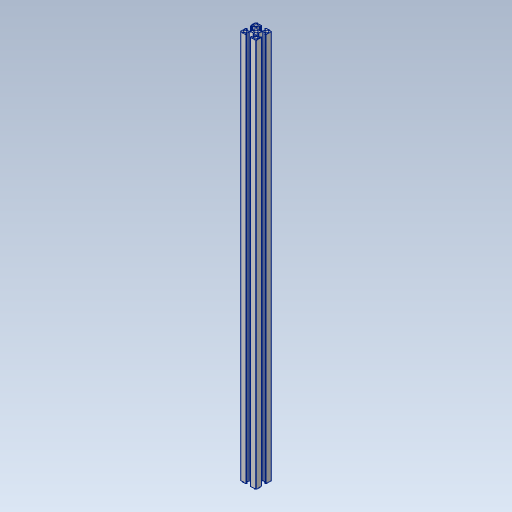
# Autodesk Inventor part: 100mm 2020
Saved by Autodesk Inventor 2021 (Build 250183000, 183)
## iProperties
Created: 2019-12-30
Part Number: 100mm 2020
Material: 알루미늄 6061
Document SubType Name: Modeling
Designer: leejun
Density: 2.7 g/cm^3
Appearance: 알루미늄 - 평지
Author: leejun
Autodesk Inventor part; units mm, degrees
ref_plane "YZ Plane" through (0, 0, 0) normal (1, 0, 0) x (0, 1, 0)
ref_plane "XZ Plane" through (0, 0, 0) normal (0, 1, 0) x (-1, 0, 0)
ref_plane "XY Plane" through (0, 0, 0) normal (0, 0, 1) x (1, 0, 0)
sketch "2020_Base" plane through (0, 0, 0) normal (0, 1, 0) x (-1, 0, 0)
  line L0 (2307.7639, 1192.1343) -> (2307.7639, 1195.3915) projected
  arc A0 (2307.7639, 1195.3915) -> (2307.4639, 1195.6915) centre (2307.4639, 1195.3915) ccw projected
  line L1 (2307.4639, 1195.6915) -> (2306.5639, 1195.6915) projected
  arc A1 (2306.2639, 1195.9915) -> (2306.5639, 1195.6915) centre (2306.5639, 1195.9915) ccw projected
  line L2 (2306.2639, 1195.9915) -> (2306.2639, 1196.8915) projected
  arc A2 (2306.5639, 1197.1915) -> (2306.2639, 1196.8915) centre (2306.5639, 1196.8915) ccw projected
  line L3 (2306.5639, 1197.1915) -> (2313.3139, 1197.1915) projected
  arc A3 (2313.6139, 1196.8915) -> (2313.3139, 1197.1915) centre (2313.3139, 1196.8915) ccw projected
  line L4 (2313.6139, 1196.8915) -> (2313.6139, 1190.1415) projected
  arc A4 (2313.3139, 1189.8415) -> (2313.6139, 1190.1415) centre (2313.3139, 1190.1415) ccw projected
  line L5 (2313.3139, 1189.8415) -> (2312.4139, 1189.8415) projected
  arc A5 (2312.1139, 1190.1415) -> (2312.4139, 1189.8415) centre (2312.4139, 1190.1415) ccw projected
  line L6 (2312.1139, 1190.1415) -> (2312.1139, 1191.0415) projected
  arc A6 (2312.1139, 1191.0415) -> (2311.8139, 1191.3415) centre (2311.8139, 1191.0415) ccw projected
  line L7 (2311.8139, 1191.3415) -> (2308.5567, 1191.3415) projected
  arc A7 (2308.5567, 1191.3415) -> (2308.3217, 1191.2281) centre (2308.5567, 1191.0415) ccw projected
  arc A8 (2308.3217, 1191.2281) -> (2306.9212, 1187.4988) centre (2313.4048, 1187.1915) ccw projected
  line L8 (2306.9212, 1187.4988) -> (2306.6139, 1187.1915) projected
  line L9 (2306.6139, 1187.1915) -> (2306.9212, 1186.8843) projected
  arc A9 (2306.9212, 1186.8843) -> (2308.3217, 1183.155) centre (2313.4048, 1187.1915) ccw projected
  arc A10 (2308.3217, 1183.155) -> (2308.5567, 1183.0415) centre (2308.5567, 1183.3415) ccw projected
  line L10 (2308.5567, 1183.0415) -> (2311.8139, 1183.0415) projected
  arc A11 (2311.8139, 1183.0415) -> (2312.1139, 1183.3415) centre (2311.8139, 1183.3415) ccw projected
  line L11 (2312.1139, 1183.3415) -> (2312.1139, 1184.2415) projected
  arc A12 (2312.4139, 1184.5415) -> (2312.1139, 1184.2415) centre (2312.4139, 1184.2415) ccw projected
  line L12 (2312.4139, 1184.5415) -> (2313.3139, 1184.5415) projected
  arc A13 (2313.6139, 1184.2415) -> (2313.3139, 1184.5415) centre (2313.3139, 1184.2415) ccw projected
  line L13 (2313.6139, 1184.2415) -> (2313.6139, 1177.4915) projected
  arc A14 (2313.3139, 1177.1915) -> (2313.6139, 1177.4915) centre (2313.3139, 1177.4915) ccw projected
  line L14 (2313.3139, 1177.1915) -> (2306.5639, 1177.1915) projected
  arc A15 (2306.2639, 1177.4915) -> (2306.5639, 1177.1915) centre (2306.5639, 1177.4915) ccw projected
  line L15 (2306.2639, 1177.4915) -> (2306.2639, 1178.3915) projected
  arc A16 (2306.5639, 1178.6915) -> (2306.2639, 1178.3915) centre (2306.5639, 1178.3915) ccw projected
  line L16 (2306.5639, 1178.6915) -> (2307.4639, 1178.6915) projected
  arc A17 (2307.4639, 1178.6915) -> (2307.7639, 1178.9915) centre (2307.4639, 1178.9915) ccw projected
  line L17 (2307.7639, 1178.9915) -> (2307.7639, 1182.2488) projected
  arc A18 (2307.7639, 1182.2488) -> (2307.6505, 1182.4837) centre (2307.4639, 1182.2488) ccw projected
  arc A19 (2307.6505, 1182.4837) -> (2303.9212, 1183.8843) centre (2303.6139, 1177.4007) ccw projected
  line L18 (2303.9212, 1183.8843) -> (2303.6139, 1184.1915) projected
  line L19 (2303.6139, 1184.1915) -> (2303.3066, 1183.8843) projected
  arc A20 (2303.3066, 1183.8843) -> (2299.5774, 1182.4837) centre (2303.6139, 1177.4007) ccw projected
  arc A21 (2299.5774, 1182.4837) -> (2299.4639, 1182.2488) centre (2299.7639, 1182.2488) ccw projected
  line L20 (2299.4639, 1182.2488) -> (2299.4639, 1178.9915) projected
  arc A22 (2299.4639, 1178.9915) -> (2299.7639, 1178.6915) centre (2299.7639, 1178.9915) ccw projected
  line L21 (2299.7639, 1178.6915) -> (2300.6639, 1178.6915) projected
  arc A23 (2300.9639, 1178.3915) -> (2300.6639, 1178.6915) centre (2300.6639, 1178.3915) ccw projected
  line L22 (2300.9639, 1178.3915) -> (2300.9639, 1177.4915) projected
  arc A24 (2300.6639, 1177.1915) -> (2300.9639, 1177.4915) centre (2300.6639, 1177.4915) ccw projected
  line L23 (2300.6639, 1177.1915) -> (2293.9139, 1177.1915) projected
  arc A25 (2293.6139, 1177.4915) -> (2293.9139, 1177.1915) centre (2293.9139, 1177.4915) ccw projected
  line L24 (2293.6139, 1177.4915) -> (2293.6139, 1184.2415) projected
  arc A26 (2293.9139, 1184.5415) -> (2293.6139, 1184.2415) centre (2293.9139, 1184.2415) ccw projected
  line L25 (2293.9139, 1184.5415) -> (2294.8139, 1184.5415) projected
  arc A27 (2295.1139, 1184.2415) -> (2294.8139, 1184.5415) centre (2294.8139, 1184.2415) ccw projected
  line L26 (2295.1139, 1184.2415) -> (2295.1139, 1183.3415) projected
  arc A28 (2295.1139, 1183.3415) -> (2295.4139, 1183.0415) centre (2295.4139, 1183.3415) ccw projected
  line L27 (2295.4139, 1183.0415) -> (2298.6712, 1183.0415) projected
  arc A29 (2298.6712, 1183.0415) -> (2298.9061, 1183.155) centre (2298.6712, 1183.3415) ccw projected
  arc A30 (2298.9061, 1183.155) -> (2300.3066, 1186.8843) centre (2293.8231, 1187.1915) ccw projected
  line L28 (2300.3066, 1186.8843) -> (2300.6139, 1187.1915) projected
  line L29 (2300.6139, 1187.1915) -> (2300.3066, 1187.4988) projected
  arc A31 (2300.3066, 1187.4988) -> (2298.9061, 1191.2281) centre (2293.8231, 1187.1915) ccw projected
  arc A32 (2298.9061, 1191.2281) -> (2298.6712, 1191.3415) centre (2298.6712, 1191.0415) ccw projected
  line L30 (2298.6712, 1191.3415) -> (2295.4139, 1191.3415) projected
  arc A33 (2295.4139, 1191.3415) -> (2295.1139, 1191.0415) centre (2295.4139, 1191.0415) ccw projected
  line L31 (2295.1139, 1191.0415) -> (2295.1139, 1190.1415) projected
  arc A34 (2294.8139, 1189.8415) -> (2295.1139, 1190.1415) centre (2294.8139, 1190.1415) ccw projected
  line L32 (2294.8139, 1189.8415) -> (2293.9139, 1189.8415) projected
  arc A35 (2293.6139, 1190.1415) -> (2293.9139, 1189.8415) centre (2293.9139, 1190.1415) ccw projected
  line L33 (2293.6139, 1190.1415) -> (2293.6139, 1196.8915) projected
  arc A36 (2293.9139, 1197.1915) -> (2293.6139, 1196.8915) centre (2293.9139, 1196.8915) ccw projected
  line L34 (2293.9139, 1197.1915) -> (2300.6639, 1197.1915) projected
  arc A37 (2300.9639, 1196.8915) -> (2300.6639, 1197.1915) centre (2300.6639, 1196.8915) ccw projected
  line L35 (2300.9639, 1196.8915) -> (2300.9639, 1195.9915) projected
  arc A38 (2300.6639, 1195.6915) -> (2300.9639, 1195.9915) centre (2300.6639, 1195.9915) ccw projected
  line L36 (2300.6639, 1195.6915) -> (2299.7639, 1195.6915) projected
  arc A39 (2299.7639, 1195.6915) -> (2299.4639, 1195.3915) centre (2299.7639, 1195.3915) ccw projected
  line L37 (2299.4639, 1195.3915) -> (2299.4639, 1192.1343) projected
  arc A40 (2299.4639, 1192.1343) -> (2299.5774, 1191.8994) centre (2299.7639, 1192.1343) ccw projected
  arc A41 (2299.5774, 1191.8994) -> (2303.3066, 1190.4988) centre (2303.6139, 1196.9824) ccw projected
  line L38 (2303.3066, 1190.4988) -> (2303.6139, 1190.1915) projected
  line L39 (2303.6139, 1190.1915) -> (2303.9212, 1190.4988) projected
  arc A42 (2303.9212, 1190.4988) -> (2307.6505, 1191.8994) centre (2303.6139, 1196.9824) ccw projected
  arc A43 (2307.6505, 1191.8994) -> (2307.7639, 1192.1343) centre (2307.4639, 1192.1343) ccw projected
  circle A44 centre (2310.6139, 1194.1915) radius 2 projected
  circle A45 centre (2303.6139, 1187.1915) radius 2.15 projected
  circle A46 centre (2296.6139, 1194.1915) radius 2 projected
  circle A47 centre (2296.6139, 1180.1915) radius 2 projected
  circle A48 centre (2310.6139, 1180.1915) radius 2 projected
  point P0 (0, 0)
extrude "500mm 2020" add sketch "2020_Base" along normal blind 500
